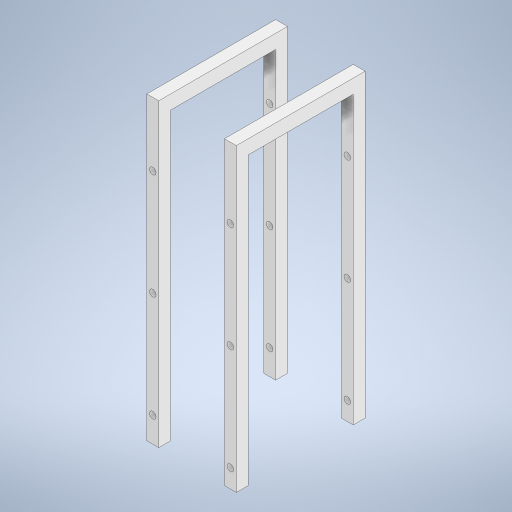
# Autodesk Inventor part: Sustentação Trilhos fixos
Saved by Autodesk Inventor 2024 (Build 280153000, 153)
## iProperties
Created: 2023-05-11
Part Number: Sustentação Trilhos fixos
Material: Plástico PET
Document SubType Name: Modeling
Designer: jpjoa
Density: 1.541 g/cm^3
Appearance: Branco
Author: jpjoa
Autodesk Inventor part; units mm, degrees
ref_plane "YZ Plane" through (0, 0, 0) normal (1, 0, 0) x (0, 1, 0)
ref_plane "XZ Plane" through (0, 0, 0) normal (0, 1, 0) x (-1, 0, 0)
ref_plane "XY Plane" through (0, 0, 0) normal (0, 0, 1) x (1, 0, 0)
sketch "Esboço1" plane through (0, 0, 0) normal (0, 1, 0) x (-1, 0, 0)
  line L0 (0, 2.7) -> (0, -2.7)
  line L1 (0, -2.7) -> (5.4, -2.7)
  line L2 (5.4, -2.7) -> (5.4, 2.7)
  line L3 (5.4, 2.7) -> (0, 2.7)
  line L4 (0, -50.353) -> (0, -55.753)
  line L5 (0, -55.753) -> (5.4, -55.753)
  line L6 (5.4, -55.753) -> (5.4, -50.353)
  line L7 (5.4, -50.353) -> (0, -50.353)
  line L8 (35.222, -50.353) -> (35.222, -55.753)
  line L9 (35.222, -55.753) -> (40.622, -55.753)
  line L10 (40.622, -55.753) -> (40.622, -50.353)
  line L11 (40.622, -50.353) -> (35.222, -50.353)
  line L12 (40.622, -2.7) -> (40.622, 2.7)
  line L13 (40.622, 2.7) -> (35.222, 2.7)
  line L14 (35.222, 2.7) -> (35.222, -2.7)
  line L15 (35.222, -2.7) -> (40.622, -2.7)
  point P0 (0, 0)
  point P1 (0, -53.053)
  point P2 (0, 0)
  point P3 (5.4, 0)
  point P4 (5.4, -53.053)
  point P5 (35.222, -53.053)
  point P6 (35.222, 0)
  point P7 (40.622, 0)
  point P8 (40.622, -53.053)
  point P9 (37.922, -55.753)
  point P10 (2.7, -55.753)
  point P11 (37.922, -2.7)
  point P12 (2.7, -2.7)
  point P13 (37.922, -50.353)
  point P14 (2.7, -50.353)
  point P15 (37.922, 2.7)
  point P16 (2.7, 2.7)
  dimension "d0" = 47.653
  dimension "d7" = 5.4
  dimension "d8" = 35.222
  constraints: 32 end point, 16 midpoint, 15 perpendicular, 4 horizontal alignment, 4 vertical, 4 vertical alignment, 2 coincident
  measures "d0" distance between parallel lines of L1 L7
  measures "d7" distance of L12.start L12.end
  measures "d8" distance of point (37.922, 2.7) point (2.7, 2.7)
extrude "Extrusão1" add sketch "Esboço1" along normal mid plane 130
sketch "Esboço3" plane through (0, 65, 0) normal (0, 1, 0) x (1, 0, 0)
  line L0 (-40.622, -2.7) -> (-35.222, -2.7) projected
  line L1 (-40.622, 55.753) -> (-35.222, 55.753) projected
  line L2 (-40.622, -2.7) -> (-40.622, 55.753)
  line L3 (-35.222, 55.753) -> (-35.222, 50.353) projected
  line L4 (-40.622, 55.753) -> (-35.222, 55.753)
  line L5 (-35.222, -2.7) -> (-35.222, 2.7) projected
  line L6 (-35.222, 55.753) -> (-35.222, -2.7)
  line L7 (-35.222, -2.7) -> (-40.622, -2.7)
  line L8 (-5.4, 55.753) -> (-5.4, 50.353) projected
  line L9 (-5.4, -2.7) -> (-5.4, 55.753)
  line L10 (0, 55.753) -> (-5.4, 55.753) projected
  line L11 (-5.4, 55.753) -> (0, 55.753)
  line L12 (-5.4, -2.7) -> (0, -2.7) projected
  line L13 (0, 55.753) -> (0, -2.7)
  line L14 (0, -2.7) -> (-5.4, -2.7)
  point P0 (0, 0)
  constraints: 16 end point, 4 perpendicular, 3 collinear, 1 vertical
extrude "Extrusão2" add sketch "Esboço3" along normal blind 6.338
sketch "Esboço4" plane through (-5.4, -65, 2.7) normal (0, 0, 1) x (1, 0, 0)
  circle A0 centre (2.7, 8.39) radius 1.5
  circle A1 centre (2.7, 56.351) radius 1.5
  circle A2 centre (2.7, 104.351) radius 1.5
  circle A3 centre (-32.522, 11.46) radius 1.5
  circle A4 centre (-32.522, 59.421) radius 1.5
  circle A5 centre (-32.522, 107.421) radius 1.5
  line L0 (5.4, 0) -> (0, 0) projected
  line L1 (-29.822, 0) -> (-35.222, 0) projected
  point P0 (5.4, 65)
  point P1 (2.7, 0)
  point P2 (-32.522, 0)
  dimension "d9" = 3
  dimension "d20" = 8.39
  dimension "d22" = 47.961
  dimension "d23" = 48
  dimension "d24" = 3.07
  dimension "d25" = 3.07
  dimension "d26" = 3.07
  constraints: 6 centre point, 6 vertical alignment, 5 equal radius, 2 midpoint
  measures "d9" diameter of A0
  measures "d20" distance from line of L0 A0.centre
  measures "d22" distance of A0.centre A1.centre
  measures "d23" distance of A1.centre A2.centre
  measures "d24" vertical distance of A2.centre A5.centre
  measures "d25" vertical distance of A0.centre A3.centre
  measures "d26" vertical distance of A1.centre A4.centre
extrude "Extrusão3" cut sketch "Esboço4" against normal up to surface (58.453 mm away)
equation "\"d8\" = Largura_trilhos"
equation "\"d9\" = Parafuso"
equation "\"d24\" = d25"
equation "\"d26\" = d25"
equation "\"Largura_trilhos\" = 35.222"
equation "\"Parafuso\" = 3"
equation "\"d11\" = 3"
equation "\"d13\" = 3"
equation "\"d15\" = 3"
equation "\"d17\" = 3"
equation "\"d19\" = 3"
